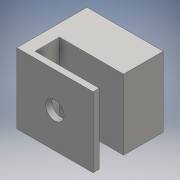
# Autodesk Inventor part: Eleveur support moteur
Saved by Autodesk Inventor 2016 (Build 200138000, 138)
## iProperties
Created: 2016-03-16
Part Number: Eleveur support moteur
Material: Generic
Document SubType Name: Modeling
Designer: Thetheos
Density: 1 g/cm^3
Appearance: Default
Author: Thetheos
Autodesk Inventor part; units mm, degrees
ref_plane "YZ Plane" through (0, 0, 0) normal (1, 0, 0) x (0, 1, 0)
ref_plane "XZ Plane" through (0, 0, 0) normal (0, 1, 0) x (-1, 0, 0)
ref_plane "XY Plane" through (0, 0, 0) normal (0, 0, 1) x (1, 0, 0)
sketch "Sketch1" plane through (0, 0, 0) normal (0, 0, 1) x (1, 0, 0)
  line L0 (0, 0) -> (25, 0)
  line L1 (25, 0) -> (25, 2)
  line L2 (25, 2) -> (4, 2)
  line L3 (4, 2) -> (4, 10)
  line L4 (4, 10) -> (25, 10)
  line L5 (25, 10) -> (25, 23)
  line L6 (25, 23) -> (0, 23)
  line L7 (0, 23) -> (0, 0)
  dimension "d0" = 25
  dimension "d1" = 2
  dimension "d2" = 8
  dimension "d5" = 13
  constraints: 16 end point, 5 perpendicular, 1 horizontal, 1 point on line, 1 vertical
  measures "d0" distance of L0.start L0.end
  measures "d1" distance of L0.end L1.end
  measures "d2" distance of L2.end L3.end
  measures "d5" distance of L4.end L5.end
extrude "Extrusion1" add sketch "Sketch1" along normal blind 23
sketch "Sketch2" plane through (0, 23, 0) normal (0, 1, 0) x (1, 0, 0)
  line L0 (0, 0) -> (25, 0) projected
  line L1 (25, 0) -> (25, -23) projected
  circle A0 centre (12.5, -11.5) radius 3
  dimension "d8" = 6
  constraints: 1 centre point
  measures "d8" diameter of A0
extrude "Extrusion2" cut sketch "Sketch2" against normal through all
body "Solid1"
